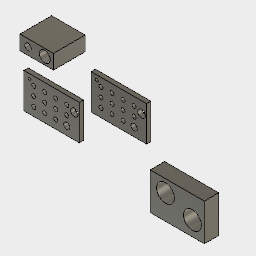
sample_model (Autodesk Fusion 360 design; units mm, degrees)
Autodesk Fusion 360 part; units mm, degrees
sketch "Sketch1" plane through (0, 0, 0) normal (0, 1, 0) x (1, 0, 0)
  line L0 (0, 0) -> (127.9417, 0)
  line L1 (127.9417, 0) -> (127.9417, -80.9687)
  line L2 (127.9417, -80.9687) -> (0, -80.9687)
  line L3 (0, -80.9687) -> (0, 0)
extrude "Extrude1" add sketch "Sketch1" along normal blind 10.2362 makes body 1
sketch "Sketch2" plane through (0, 0, 0) normal (0, 1, 0) x (1, 0, 0)
  circle A0 centre (22.9713, -19.6698) radius 4.6491
  circle A1 centre (48.3713, -19.6698) radius 4.6491
  circle A2 centre (73.7713, -19.6698) radius 4.6491
  circle A3 centre (99.1713, -19.6698) radius 4.6491
  circle A4 centre (22.9713, -40.701) radius 4.6491
  circle A5 centre (48.3713, -40.701) radius 4.6491
  circle A6 centre (73.7713, -40.701) radius 4.6491
  circle A7 centre (99.1713, -40.701) radius 4.6491
  circle A8 centre (22.9713, -61.7322) radius 4.6491
  circle A9 centre (48.3713, -61.7322) radius 4.6491
  circle A10 centre (73.7713, -61.7322) radius 4.6491
  circle A11 centre (99.1713, -61.7322) radius 4.6491
  dimension "d5" = 76.2
  dimension "d6" = -42.0624
extrude "Extrude2" cut sketch "Sketch2" along normal blind 27.7114 bodies 1
copy_body "Body->Comp1" bodies 1 removing the originals makes body 2 in component "Component"
move_face "OffsetFaces1" offset -2.54 1 faces at (103.7974, 6.8241, 19.2069) on bodies 2 in component "Component"
sketch "Sketch3" plane through (0, 0, 0) normal (0, -1, 0) x (1, 0, 0)
  circle A0 centre (203.3425, 94.8052) radius 4.6491
  circle A1 centre (254.1425, 94.8052) radius 7.1891
  circle A2 centre (203.3425, 136.8676) radius 4.6491
  circle A3 centre (228.7425, 136.8676) radius 4.6491
  circle A4 centre (228.7425, 94.8052) radius 4.6491
  circle A5 centre (177.9425, 94.8052) radius 4.6491
  circle A6 centre (203.3425, 115.8364) radius 4.6491
  circle A7 centre (254.1425, 115.8364) radius 4.6491
  circle A8 centre (177.9425, 136.8676) radius 4.6491
  circle A9 centre (254.1425, 136.8676) radius 4.6491
  circle A10 centre (228.7425, 115.8364) radius 4.6491
  circle A11 centre (177.9425, 115.8364) radius 4.6491
  line L0 (282.9128, 156.1041) -> (154.9711, 156.1041)
  line L1 (154.9711, 156.1041) -> (154.9711, 75.1354)
  line L2 (154.9711, 75.1354) -> (282.9128, 75.1354)
  line L3 (282.9128, 75.1354) -> (282.9128, 156.1041)
  circle A12 centre (168.2289, 145.5598) radius 3.384
  circle A13 centre (271.4044, 130.3705) radius 8.5468
extrude "Extrude1'" cut sketch "Sketch3" against normal blind 31.3436 contours A12 | A13 sketch seen with x (1, 0, 0) y (0, 1, 0) z (0, 0, 1) at (-154.9711, 0, -75.1354) bodies 2 in component "Component"
sketch "Sketch1 (2)" plane through (0, 0, 0) normal (0, 1, 0) x (1, 0, 0) in component "Component'"
  line L0 (-9.2161, -149.1619) -> (68.306, -149.1619)
  line L1 (68.306, -149.1619) -> (68.306, -115.5159)
  line L2 (68.306, -115.5159) -> (-9.2161, -115.5159)
  line L3 (-9.2161, -115.5159) -> (-9.2161, -149.1619)
  circle A0 centre (9.883, -132.7089) radius 7.421
  circle A1 centre (48.2856, -132.7089) radius 12.6162
extrude "Extrude1''" add sketch "Sketch1 (2)" along normal blind 73.3806 separate body makes body 3 in component "Component'"
sketch "Sketch4" plane through (0, 0, 0) normal (0, 1, 0) x (1, 0, 0)
  line L0 (291.1513, -28.1062) -> (416.1443, -28.1062)
  line L1 (416.1443, -28.1062) -> (416.1443, 57.383)
  line L2 (416.1443, 57.383) -> (291.1513, 57.383)
  line L3 (291.1513, 57.383) -> (291.1513, -28.1062)
  circle A0 centre (326.4438, 0.3255) radius 20.5105
  circle A1 centre (388.7017, 23.4153) radius 20.5105
extrude "Extrude3" add sketch "Sketch4" along normal blind 33.5 separate body makes body 4
component "Component" placed x (1, 0, 0) y (0, 1, 0) z (0, 0, 1) at (0, 0, 0)
component "Component" placed x (1, 0, 0) y (0, 1, 0) z (0, 0, 1) at (154.9711, 0, 75.1354)
component "Component'" placed x (1, 0, 0) y (0, 1, 0) z (0, 0, 1) at (0, 0, 0)
